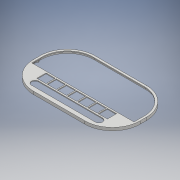
# Autodesk Inventor part: Game_ColoniesV2
Saved by Autodesk Inventor 2018 (Build 220112000, 112)
## iProperties
Created: 2021-04-22
Part Number: Game_ColoniesV2
Material: Generic
Document SubType Name: Modeling
Designer: Bradley
Density: 1 g/cm^3
Appearance: Default
Author: Bradley
Autodesk Inventor part; units mm, degrees
ref_plane "YZ Plane" through (0, 0, 0) normal (1, 0, 0) x (0, 1, 0)
ref_plane "XZ Plane" through (0, 0, 0) normal (0, 1, 0) x (-1, 0, 0)
ref_plane "XY Plane" through (0, 0, 0) normal (0, 0, 1) x (1, 0, 0)
sketch "Sketch1" plane through (0, 0, 0) normal (0, 0, 1) x (1, 0, 0)
  line L0 (-25, -30) -> (25, -30)
  line L1 (52, -3) -> (52, 3)
  line L2 (25, 30) -> (-25, 30)
  line L3 (-52, 3) -> (-52, -3)
  line L4 (-52, -30) -> (52, 30) construction
  line L5 (52, -30) -> (-52, 30) construction
  arc A0 (-25, 30) -> (-52, 3) centre (-25, 3) ccw
  arc A1 (52, 3) -> (25, 30) centre (25, 3) ccw
  arc A2 (25, -30) -> (52, -3) centre (25, -3) ccw
  arc A3 (-52, -3) -> (-25, -30) centre (-25, -3) ccw
  line L6 (-51.1, 3) -> (-51.1, -3)
  arc A4 (-51.1, -3) -> (-25, -29.1) centre (-25, -3) ccw
  line L7 (-25, -29.1) -> (25, -29.1)
  arc A5 (25, -29.1) -> (51.1, -3) centre (25, -3) ccw
  line L8 (51.1, -3) -> (51.1, 3)
  arc A6 (51.1, 3) -> (25, 29.1) centre (25, 3) ccw
  line L9 (25, 29.1) -> (-25, 29.1)
  arc A7 (-25, 29.1) -> (-51.1, 3) centre (-25, 3) ccw
  line L10 (-25, 28) -> (25, 28)
  arc A8 (50, 3) -> (25, 28) centre (25, 3) ccw
  line L11 (50, 3) -> (50, -7)
  line L12 (-50, -7) -> (-50, 3)
  arc A9 (-25, 28) -> (-50, 3) centre (-25, 3) ccw
  line L13 (-50, -7) -> (50, -7)
  line L14 (-34.5, -8.5) -> (-25.5, -8.5)
  line L15 (-25.5, -8.5) -> (-25.5, -17.5)
  line L16 (-25.5, -17.5) -> (-34.5, -17.5)
  line L17 (-34.5, -17.5) -> (-34.5, -8.5)
  line L18 (-24.5, -8.5) -> (-15.5, -8.5)
  line L19 (-24.5, -17.5) -> (-24.5, -8.5)
  line L20 (-15.5, -8.5) -> (-15.5, -17.5)
  line L21 (-15.5, -17.5) -> (-24.5, -17.5)
  line L22 (-14.5, -8.5) -> (-5.5, -8.5)
  line L23 (-14.5, -17.5) -> (-14.5, -8.5)
  line L24 (-5.5, -8.5) -> (-5.5, -17.5)
  line L25 (-5.5, -17.5) -> (-14.5, -17.5)
  line L26 (-4.5, -8.5) -> (4.5, -8.5)
  line L27 (-4.5, -17.5) -> (-4.5, -8.5)
  line L28 (4.5, -8.5) -> (4.5, -17.5)
  line L29 (4.5, -17.5) -> (-4.5, -17.5)
  line L30 (5.5, -8.5) -> (14.5, -8.5)
  line L31 (5.5, -17.5) -> (5.5, -8.5)
  line L32 (14.5, -8.5) -> (14.5, -17.5)
  line L33 (14.5, -17.5) -> (5.5, -17.5)
  line L34 (15.5, -8.5) -> (24.5, -8.5)
  line L35 (15.5, -17.5) -> (15.5, -8.5)
  line L36 (24.5, -8.5) -> (24.5, -17.5)
  line L37 (24.5, -17.5) -> (15.5, -17.5)
  line L38 (25.5, -8.5) -> (34.5, -8.5)
  line L39 (25.5, -17.5) -> (25.5, -8.5)
  line L40 (34.5, -8.5) -> (34.5, -17.5)
  line L41 (34.5, -17.5) -> (25.5, -17.5)
  line L42 (-31.25, -22.5) -> (31.25, -22.5) construction
  line L43 (-31.25, -26) -> (31.25, -26)
  line L44 (31.25, -19) -> (-31.25, -19)
  arc A10 (-31.25, -19) -> (-31.25, -26) centre (-31.25, -22.5) ccw
  arc A11 (31.25, -26) -> (31.25, -19) centre (31.25, -22.5) ccw
  point P0 (0, 0)
  point P1 (0, -22.5)
  point P2 (0, 0)
  point P3 (0, -8.5)
  point P4 (4.5, -13)
  point P5 (0, 0)
  dimension "d0" = 104
  dimension "d1" = 60
  dimension "d2" = 27
  dimension "d3" = 58.2
  dimension "d4" = 2
  dimension "d5" = 23
  dimension "d6" = 9
  dimension "d9" = 10
  dimension "d16" = 62.5
  dimension "d17" = 7
  dimension "d24" = 13
  dimension "d25" = 22.5
  constraints: 92 end point, 24 point on circle, 13 tangent, 12 centre point, 8 parallel, 8 point on line, 7 midpoint, 5 horizontal, 4 perpendicular, 3 equal radius, 2 vertical alignment, 58 other
  measures "d0" distance of L5.end L4.end
  measures "d1" distance of L4.end L5.start
  measures "d2" radius of A0
  measures "d3" distance between parallel lines of L7 L9
  measures "d4" distance between parallel lines of L2 L10
  measures "d5" distance between parallel lines of L0 L13
  measures "d6" distance of L15.end L16.end
  measures "d9" distance of L14.start L18.start
  measures "d16" distance of L42.start L42.end
  measures "d17" diameter of A11
  measures "d24" vertical distance of point (0, 0) point (4.5, -13)
  measures "d25" distance of point (0, -22.5) point (0, 0)
extrude "Extrusion1" add sketch "Sketch1" against normal blind 2.1 contours A3 L3 A0 L2 A1 L1 A2 L0
extrude "Extrusion2" add sketch "Sketch1" along normal blind 0.8 contours A3 L3 A0 L2 A1 L1 A2 L0 | A7 L9 A6 L8 A5 L7 A4 L6
sketch "Sketch2" plane through (0, 0, -2.1) normal (0, 0, -1) x (-1, 0, 0)
  arc A0 (25, -29.1) -> (51.1, -3) centre (25, -3) ccw projected
  line L0 (25, -29.1) -> (-25, -29.1) projected
  arc A1 (-51.1, -3) -> (-25, -29.1) centre (-25, -3) ccw projected
  line L1 (-51.1, -3) -> (-51.1, 3) projected
  arc A2 (-25, 29.1) -> (-51.1, 3) centre (-25, 3) ccw projected
  line L2 (-25, 29.1) -> (25, 29.1) projected
  arc A3 (51.1, 3) -> (25, 29.1) centre (25, 3) ccw projected
  line L3 (51.1, 3) -> (51.1, -3) projected
  line L4 (25, 30) -> (-25, 30) projected
  arc A4 (-25, 30) -> (-52, 3) centre (-25, 3) ccw projected
  line L5 (-52, 3) -> (-52, -3) projected
  arc A5 (-52, -3) -> (-25, -30) centre (-25, -3) ccw projected
  line L6 (-25, -30) -> (25, -30) projected
  arc A6 (25, -30) -> (52, -3) centre (25, -3) ccw projected
  line L7 (52, -3) -> (52, 3) projected
  arc A7 (52, 3) -> (25, 30) centre (25, 3) ccw projected
  line L8 (51.1, 3) -> (51.1, -3) projected
  line L9 (51.1, -1.7321) -> (50.1, 0)
  line L10 (50.1, 0) -> (51.1, 1.7321)
  point P0 (0, 0)
  point P1 (51.1, 0)
  dimension "d26" = 1
  dimension "d27" = 120
  constraints: 4 end point, 2 point on line, 1 equal length, 1 horizontal alignment, 1 midpoint
  measures "d26" distance from line of L9.end L3
  measures "d27" angle of L10 L9
extrude "Extrusion3" add sketch "Sketch2" against normal up to surface (2.1 mm away) contours L9 L10 L3
mirror "Mirror1" about plane through (0, 0, 0) normal (1, 0, 0) of "Extrusion3"
body "Solid1"
